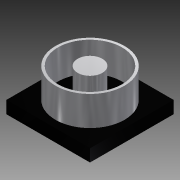
# Autodesk Inventor part: MICRO-SMA
Saved by Autodesk Inventor 2015 SP1 (Build 190203100, 203)
## iProperties
Created: 2015-10-19
Part Number: MICRO-SMA
Material: Generic
Document SubType Name: Modeling
Designer: Kartikye
Density: 1 g/cm^3
Appearance: MICRO-SMA, MICRO-SMA
Author: Kartikye
Autodesk Inventor part; units mm, degrees
ref_plane "YZ Plane" through (0, 0, 0) normal (1, 0, 0) x (0, 1, 0)
ref_plane "XZ Plane" through (0, 0, 0) normal (0, 1, 0) x (-1, 0, 0)
ref_plane "XY Plane" through (0, 0, 0) normal (0, 0, 1) x (1, 0, 0)
sketch "MICRO-SMA, MICRO-SMA_13" plane through (0, 0, 0) normal (0, 0, 1) x (1, 0, 0)
  line L0 (-0.85, -0.85) -> (0.85, -0.85)
  line L1 (0.85, -0.85) -> (0.85, 0.85)
  line L2 (0.85, 0.85) -> (-0.85, 0.85)
  line L3 (-0.85, 0.85) -> (-0.85, -0.85)
  line L4 (-0.85, -0.85) -> (0.85, 0.85) construction
  line L5 (0.85, -0.85) -> (-0.85, 0.85) construction
  point P0 (0, 0)
  dimension "d4" = 1.7
  dimension "d5" = 1.7
  constraints: 12 end point, 2 midpoint, 2 parallel, 1 horizontal, 1 perpendicular
  measures "d4" distance of L2.end L1.end
  measures "d5" distance of L1.end L0.end
extrude "Extrusion1" add sketch "MICRO-SMA, MICRO-SMA_13" along normal blind 0.25
sketch "Sketch2" plane through (0, 0, 0.25) normal (0, 0, 1) x (1, 0, 0)
  circle A0 centre (0, 0) radius 0.7
  circle A1 centre (0, 0) radius 0.65
  circle A2 centre (0, 0) radius 0.25
  dimension "d6" = 1.4
  dimension "d7" = 1.3
  dimension "d8" = 0.5
  constraints: 3 centre point, 3 coincident
  measures "d6" diameter of A0
  measures "d7" diameter of A1
  measures "d8" diameter of A2
extrude "Extrusion2" add sketch "Sketch2" along normal blind 0.6
body "Solid1"
